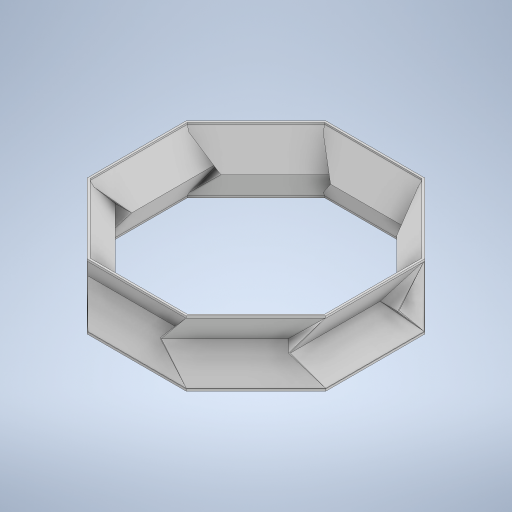
# Autodesk Inventor part: 팔각형 OV-PAM 층 한개
Saved by Autodesk Inventor 2024 (Build 280153000, 153)
## iProperties
Created: 2023-06-16
Part Number: 팔각형 OV-PAM 층 한개
Material: 일반
Document SubType Name: Modeling
Designer: jsw
Density: 1 g/cm^3
Appearance: 기본값
Author: jsw
Autodesk Inventor part; units mm, degrees
ref_plane "YZ Plane" through (0, 0, 0) normal (1, 0, 0) x (0, 1, 0)
ref_plane "XZ Plane" through (0, 0, 0) normal (0, 1, 0) x (-1, 0, 0)
ref_plane "XY Plane" through (0, 0, 0) normal (0, 0, 1) x (1, 0, 0)
sketch "스케치1" plane through (0, 0, 0) normal (0, 1, 0) x (-1, 0, 0)
  line L0 (-46.0919, 19.0919) -> (-19.0919, 46.0919)
  line L1 (-19.0919, 46.0919) -> (19.0919, 46.0919)
  line L2 (19.0919, 46.0919) -> (46.0919, 19.0919)
  line L3 (46.0919, 19.0919) -> (46.0919, -19.0919)
  line L4 (46.0919, -19.0919) -> (19.0919, -46.0919)
  line L5 (19.0919, -46.0919) -> (-19.0919, -46.0919)
  line L6 (-19.0919, -46.0919) -> (-46.0919, -19.0919)
  line L7 (-46.0919, -19.0919) -> (-46.0919, 19.0919)
  line L8 (-19.3404, 46.6919) -> (19.3404, 46.6919)
  line L9 (19.3404, 46.6919) -> (46.6919, 19.3404)
  line L10 (46.6919, 19.3404) -> (46.6919, -19.3404)
  line L11 (46.6919, -19.3404) -> (19.3404, -46.6919)
  line L12 (19.3404, -46.6919) -> (-19.3404, -46.6919)
  line L13 (-19.3404, -46.6919) -> (-46.6919, -19.3404)
  line L14 (-46.6919, -19.3404) -> (-46.6919, 19.3404)
  line L15 (-46.6919, 19.3404) -> (-19.3404, 46.6919)
  point P0 (0, 0)
  point P1 (0, 0)
  point P2 (0, 0)
  dimension "d0" = 38.1838
  dimension "d2" = 0.6
  constraints: 32 end point, 2 coincident, 2 horizontal, 34 other
  measures "d0" distance of L0.end L1.end
  measures "d2" distance between parallel lines of L10 L3
extrude "돌출2" add sketch "스케치1" along normal blind 12 contours L0 L1 L2 L3 L4 L5 L6 L7 | L8 L9 L10 L11 L12 L13 L14 L15
ref_plane "작업 평면2" through (46.6919, 0, 19.3404) normal (-0.8660254, -0.5, 0) x (0, 0, -1)
sketch "스케치3" plane through (46.6919, 0, 19.3404) normal (1, 0, 0) x (0, 0, -1)
  line L0 (0, 0) -> (0, 12) projected
  line L1 (0, 12) -> (38.6808, 12) projected
  line L2 (0, 0) -> (38.6808, 0)
  line L3 (38.6808, 0) -> (38.6808, 12)
  line L4 (38.6808, 12) -> (0, 12)
  line L5 (0, 12) -> (0, 0)
  line L6 (0, 12) -> (-7.3047, 12)
  line L7 (-27.3515, 12) -> (0, 12) projected
  line L8 (0, 0) -> (-7.3047, 12)
  line L9 (38.6808, 12) -> (19.3404, 12)
  line L10 (28.3404, 12) -> (38.6808, 0)
  point P0 (19.3404, 0)
  dimension "d17" = 121.33
  dimension "d49" = 9
  constraints: 16 end point, 5 midpoint, 2 parallel, 2 point on line, 1 horizontal, 1 perpendicular
  measures "d17" angle of L8 L2
  measures "d49" distance of point (19.34, 12) L10.start
extrude "돌출4" cut sketch "스케치3" against normal up to surface contours L8 L6 L0 | L0 L1 L10 L2 surface through (46.6919, 0, 19.3404) normal (-0.8660254, -0.5, 0)
pattern_circular "원형 패턴1" count 8 over 360 about axis through (0, -10, 0) along (0, 1, 0) of "돌출4"
mirror "미러5" about plane through (0, 12, 0) normal (0, 1, 0) of "돌출2", "돌출4", "원형 패턴1"
sketch "스케치9" plane through (-19.3404, 24, -46.6919) normal (0, 1, 0) x (1, 0, 0)
  line L0 (66.0323, -66.0323) -> (66.0323, -27.3515) projected
  line L1 (66.0323, -27.3515) -> (38.6808, 0) projected
  line L2 (38.6808, 0) -> (0, 0) projected
  line L3 (0, 0) -> (-27.3515, -27.3515) projected
  line L4 (-27.3515, -27.3515) -> (-27.3515, -66.0323) projected
  line L5 (-27.3515, -66.0323) -> (0, -93.3838) projected
  line L6 (0, -93.3838) -> (38.6808, -93.3838) projected
  line L7 (38.6808, -93.3838) -> (66.0323, -66.0323) projected
  point P0 (19.3404, -46.6919)
extrude "돌출8" add sketch "스케치9" along normal blind 0.8
sketch "스케치10" plane through (0, 0, 0) normal (0, -1, 0) x (1, 0, 0)
  line L0 (46.6919, 19.3404) -> (46.6919, -19.3404) projected
  line L1 (19.3404, 46.6919) -> (46.6919, 19.3404) projected
  line L2 (-19.3404, 46.6919) -> (19.3404, 46.6919) projected
  line L3 (-46.6919, 19.3404) -> (-19.3404, 46.6919) projected
  line L4 (-46.6919, -19.3404) -> (-46.6919, 19.3404) projected
  line L5 (-19.3404, -46.6919) -> (-46.6919, -19.3404) projected
  line L6 (19.3404, -46.6919) -> (-19.3404, -46.6919) projected
  line L7 (46.6919, -19.3404) -> (19.3404, -46.6919) projected
  point P0 (0, 0)
extrude "돌출9" add sketch "스케치10" along normal blind 0.8
shell "쉘6" thickness 0.6 removed faces 2 at (6.4468, 24.8, -2.6704) at (6.4468, -0.8, 2.6704)
sketch "스케치12" plane through (-19.3404, 24.8, -46.6919) normal (0, 1, 0) x (1, 0, 0)
  line L0 (-0.0828, 0.2) -> (38.7637, 0.2)
  line L1 (38.7637, 0.2) -> (66.2323, -27.2686)
  line L2 (66.2323, -27.2686) -> (66.2323, -66.1151)
  line L3 (66.2323, -66.1151) -> (38.7637, -93.5838)
  line L4 (38.7637, -93.5838) -> (-0.0828, -93.5838)
  line L5 (-0.0828, -93.5838) -> (-27.5515, -66.1151)
  line L6 (-27.5515, -66.1151) -> (-27.5515, -27.2686)
  line L7 (-27.5515, -27.2686) -> (-0.0828, 0.2)
  line L8 (66.0323, -66.0323) -> (66.0323, -27.3515) projected
  line L9 (0, -93.3838) -> (38.6808, -93.3838) projected
  line L10 (38.4323, -92.7838) -> (0.2485, -92.7838) projected
  line L11 (65.4323, -27.6) -> (65.4323, -65.7838) projected
  line L12 (65.4323, -65.7838) -> (38.4323, -92.7838) projected
  line L13 (38.4323, -92.7838) -> (0.2485, -92.7838) projected
  line L14 (0.2485, -92.7838) -> (-26.7515, -65.7838) projected
  line L15 (-26.7515, -65.7838) -> (-26.7515, -27.6) projected
  line L16 (-26.7515, -27.6) -> (0.2485, -0.6) projected
  line L17 (0.2485, -0.6) -> (38.4323, -0.6) projected
  line L18 (38.4323, -0.6) -> (65.4323, -27.6) projected
  line L19 (66.0323, -27.3515) -> (38.6808, 0) projected
  line L20 (38.6808, 0) -> (0, 0) projected
  line L21 (0, 0) -> (-27.3515, -27.3515) projected
  line L22 (-27.3515, -27.3515) -> (-27.3515, -66.0323) projected
  line L23 (-27.3515, -66.0323) -> (0, -93.3838) projected
  line L24 (0, -93.3838) -> (38.6808, -93.3838) projected
  line L25 (38.6808, -93.3838) -> (66.0323, -66.0323) projected
  line L26 (66.0323, -66.0323) -> (66.0323, -27.3515) projected
  point P0 (19.3404, -46.6919)
  point P1 (19.3404, -46.6919)
  point P2 (0, -93.3838)
  dimension "d50" = 0.2
  constraints: 16 end point, 1 coincident, 1 horizontal, 17 other
  measures "d50" distance between parallel lines of L8 L2
extrude "돌출10" add sketch "스케치12" against normal blind 0.8 contours L0 L1 L2 L3 L4 L5 L6 L7
ref_plane "작업 평면6" through (-19.3404, 12, -46.6919) normal (0, 1, 0) x (1, 0, 0)
mirror "미러8" about plane through (-19.3404, 12, -46.6919) normal (0, 1, 0) of "돌출10"
